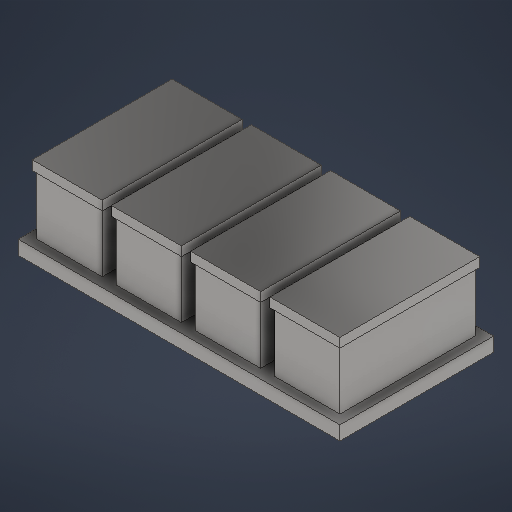
# Autodesk Inventor part: SACMI PH1500 30X60 DIE SET TILES BOTTOM MOLD
Saved by Autodesk Inventor 2025 (Build 290162000, 162)
## iProperties
Created: 2024-05-02
Part Number: SACMI PH1500 30X60 DIE SET TILES BOTTOM MOLD
Material: Generic
Document SubType Name: Modeling
Designer: zulet
Density: 1 g/cm^3
Appearance: Steel - Polished
Author: zulet
Autodesk Inventor part; units mm, degrees
ref_plane "YZ Plane" through (0, 0, 0) normal (1, 0, 0) x (0, 1, 0)
ref_plane "XZ Plane" through (0, 0, 0) normal (0, 1, 0) x (-1, 0, 0)
ref_plane "XY Plane" through (0, 0, 0) normal (0, 0, 1) x (1, 0, 0)
sketch "Sketch1" plane through (0, 0, 0) normal (0, 1, 0) x (-1, 0, 0)
  line L0 (-690, -330) -> (690, -330)
  line L1 (690, -330) -> (690, 330)
  line L2 (690, 330) -> (-690, 330)
  line L3 (-690, 330) -> (-690, -330)
  line L4 (-690, -330) -> (690, 330) construction
  line L5 (690, -330) -> (-690, 330) construction
  point P0 (0, 0)
  dimension "d0" = 1380
  dimension "d1" = 660
  constraints: 12 end point, 2 midpoint, 2 parallel, 1 horizontal, 1 perpendicular
  measures "d0" distance of L2.end L1.end
  measures "d1" distance of L1.end L0.end
extrude "Extrusion1" add sketch "Sketch1" along normal blind 60
sketch "Sketch2" plane through (0, 60, 0) normal (0, 1, 0) x (1, 0, 0)
  line L0 (-660, 300) -> (-360, 300) construction
  line L1 (-360, 300) -> (-360, -300) construction
  line L2 (-360, -300) -> (-660, -300) construction
  line L3 (-660, -300) -> (-660, 300) construction
  line L4 (-660, 300) -> (-360, -300) construction
  line L5 (-360, 300) -> (-660, -300) construction
  line L6 (-690, 330) -> (-690, -330) projected
  line L7 (-690, 0) -> (690, 0) construction
  line L8 (690, -330) -> (690, 330) construction
  line L9 (-370, 290) -> (-650, 290)
  line L10 (-650, 290) -> (-650, -290)
  line L11 (-650, -290) -> (-370, -290)
  line L12 (-370, -290) -> (-370, 290)
  line L13 (-20, 300) -> (-20, -300) construction
  line L14 (-30, -290) -> (-30, 290)
  line L15 (-30, 290) -> (-310, 290)
  line L16 (-320, 300) -> (-20, 300) construction
  line L17 (-310, 290) -> (-310, -290)
  line L18 (-320, -300) -> (-320, 300) construction
  line L19 (-320, 300) -> (-20, -300) construction
  line L20 (-20, 300) -> (-320, -300) construction
  line L21 (-310, -290) -> (-30, -290)
  line L22 (-20, -300) -> (-320, -300) construction
  line L23 (320, 300) -> (320, -300) construction
  line L24 (310, -290) -> (310, 290)
  line L25 (310, 290) -> (30, 290)
  line L26 (20, 300) -> (320, 300) construction
  line L27 (30, 290) -> (30, -290)
  line L28 (20, -300) -> (20, 300) construction
  line L29 (20, 300) -> (320, -300) construction
  line L30 (320, 300) -> (20, -300) construction
  line L31 (30, -290) -> (310, -290)
  line L32 (320, -300) -> (20, -300) construction
  line L33 (660, 300) -> (660, -300) construction
  line L34 (650, -290) -> (650, 290)
  line L35 (650, 290) -> (370, 290)
  line L36 (360, 300) -> (660, 300) construction
  line L37 (370, 290) -> (370, -290)
  line L38 (360, -300) -> (360, 300) construction
  line L39 (360, 300) -> (660, -300) construction
  line L40 (660, 300) -> (360, -300) construction
  line L41 (370, -290) -> (650, -290)
  line L42 (660, -300) -> (360, -300) construction
  point P0 (0, 0)
  point P1 (-510, 0)
  point P2 (-170, 0)
  point P3 (170, 0)
  point P4 (510, 0)
  dimension "d4" = 300
  dimension "d5" = 600
  dimension "d6" = 30
  dimension "d7" = 10
  dimension "d10" = 340
  constraints: 82 end point, 4 midpoint, 4 parallel, 2 horizontal, 2 perpendicular, 1 point on line, 60 other
  measures "d4" distance of L1.end L2.end
  measures "d5" distance of L0.end L1.end
  measures "d6" distance between parallel lines of L6 L3
  measures "d7" distance between parallel lines of L0 L9
  measures "d10" distance of L0.end L13.start
extrude "Extrusion2" add sketch "Sketch2" along normal blind 255
sketch "Sketch3" plane through (0, 315, 0) normal (0, 1, 0) x (1, 0, 0)
  line L0 (-650, 290) -> (-650, -290) construction
  line L1 (-650, -290) -> (-370, -290) construction
  line L2 (-370, -290) -> (-370, 290) construction
  line L3 (-370, 290) -> (-650, 290) construction
  line L4 (-30, 290) -> (-310, 290) construction
  line L5 (-310, 290) -> (-310, -290) construction
  line L6 (-310, -290) -> (-30, -290) construction
  line L7 (-30, -290) -> (-30, 290) construction
  line L8 (310, 290) -> (30, 290) construction
  line L9 (30, 290) -> (30, -290) construction
  line L10 (30, -290) -> (310, -290) construction
  line L11 (310, -290) -> (310, 290) construction
  line L12 (650, 290) -> (370, 290) construction
  line L13 (370, 290) -> (370, -290) construction
  line L14 (370, -290) -> (650, -290) construction
  line L15 (650, -290) -> (650, 290) construction
  line L16 (-360, 300) -> (-360, -300)
  line L17 (-360, -300) -> (-660, -300)
  line L18 (-660, -300) -> (-660, 300)
  line L19 (-660, 300) -> (-360, 300)
  line L20 (-20, 300) -> (-320, 300)
  line L21 (-320, 300) -> (-320, -300)
  line L22 (-320, -300) -> (-20, -300)
  line L23 (-20, -300) -> (-20, 300)
  line L24 (20, 300) -> (320, 300)
  line L25 (320, 300) -> (320, -300)
  line L26 (320, -300) -> (20, -300)
  line L27 (20, -300) -> (20, 300)
  line L28 (360, -300) -> (360, 300)
  line L29 (360, 300) -> (660, 300)
  line L30 (660, 300) -> (660, -300)
  line L31 (660, -300) -> (360, -300)
  point P0 (0, 0)
  dimension "d17" = 10
  dimension "d18" = 10
  dimension "d19" = 10
  dimension "d20" = 10
  constraints: 32 end point, 12 other
  measures "d17" distance between parallel lines of L2 L16
  measures "d18" distance between parallel lines of L7 L23
  measures "d19" distance between parallel lines of L8 L24
  measures "d20" distance between parallel lines of L13 L28
extrude "Extrusion3" add sketch "Sketch3" along normal blind 40
sketch "Sketch4" plane through (0, 0, 0) normal (0, -1, 0) x (1, 0, 0)
  circle A0 centre (-200, 0) radius 50
  circle A1 centre (200, 0) radius 50
  line L0 (-200, 0) -> (200, 0) construction
  point P0 (0, 0)
  point P1 (0, 0)
  dimension "d23" = 100
  dimension "d24" = 100
  dimension "d25" = 400
  constraints: 2 centre point, 2 end point, 1 coincident, 1 horizontal, 1 midpoint
  measures "d23" diameter of A0
  measures "d24" diameter of A1
  measures "d25" distance of L0.start L0.end
extrude "Extrusion4" cut sketch "Sketch4" against normal blind 80
body "Solid1"
